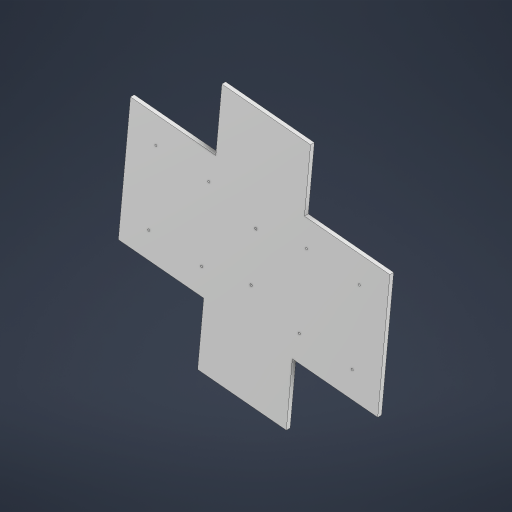
# Autodesk Inventor part: Pod_Holders
Saved by Autodesk Inventor 2024.2 (Build 282272000, 272)
## iProperties
Created: 2024-03-31
Part Number: Pod_Holders
Material: Aluminum
Document SubType Name: Modeling
Designer: warm
Density: 2.7 g/cm^3
Appearance: Satin
Mass: 2143.16 g
Surface Area: 2616.28 cm^2
Volume: 793.761 cm^3
Author: warm
Autodesk Inventor part; units mm, degrees
ref_plane "YZ Plane" through (0, 0, 0) normal (1, 0, 0) x (0, 1, 0)
ref_plane "XZ Plane" through (0, 0, 0) normal (0, 1, 0) x (-1, 0, 0)
sketch "Sketch1" plane through (0, 0, 0) normal (0, 0, 1) x (1, 0, 0)
  line L0 (-65.7194, 60.3542) -> (-75.7574, -47.1434) projected
  line L1 (-75.7574, -47.1434) -> (65.7194, -60.3542) projected
  line L2 (-95.8276, -262.0778) -> (45.6492, -275.2887) projected
  line L3 (-105.8656, -369.5754) -> (-95.8276, -262.0778) projected
  line L4 (-212.6955, 74.0786) -> (-222.7334, -33.419) projected
  line L5 (-222.7334, -33.419) -> (-364.2102, -20.2081) projected
  line L6 (-242.8036, -248.3534) -> (-384.2805, -235.1426) projected
  line L7 (-252.8416, -355.851) -> (-242.8036, -248.3534) projected
  circle A0 centre (-72.4386, -92.2695) radius 2.6 construction
  circle A1 centre (-84.3392, -219.7151) radius 2.6 construction
  circle A2 centre (3.2796, -227.8968) radius 2.6 construction
  circle A3 centre (15.1803, -100.4512) radius 2.6 construction
  circle A4 centre (-156.3158, -105.5656) radius 1.7526 construction
  circle A5 centre (-164.2553, -190.5905) radius 1.7526 construction
  circle A6 centre (-246.2503, -204.5961) radius 2.6 construction
  circle A7 centre (-333.8691, -196.4144) radius 2.6 construction
  circle A8 centre (-321.9685, -68.9688) radius 2.6 construction
  circle A9 centre (-234.3496, -77.1505) radius 2.6 construction
  circle A10 centre (15.1803, -100.4512) radius 1.6
  circle A11 centre (3.2796, -227.8968) radius 1.6
  circle A12 centre (-84.3392, -219.7151) radius 1.6
  circle A13 centre (-72.4386, -92.2695) radius 1.6
  circle A14 centre (-234.3496, -77.1505) radius 1.6
  circle A15 centre (-321.9685, -68.9688) radius 1.6
  circle A16 centre (-333.8691, -196.4144) radius 1.6
  circle A17 centre (-246.2503, -204.5961) radius 1.6
  line L8 (-65.7194, 60.3542) -> (-212.6955, 74.0786)
  line L9 (-364.2102, -20.2081) -> (-384.2805, -235.1426)
  line L10 (-252.8416, -355.851) -> (-105.8656, -369.5754)
  line L11 (45.6492, -275.2887) -> (65.7194, -60.3542)
  circle A18 centre (-156.3158, -105.5656) radius 1.8288
  circle A19 centre (-164.2553, -190.5905) radius 1.8288
  point P0 (0, 0)
  dimension "d0" = 3.2
  dimension "d1" = 3.2
  dimension "d2" = 3.2
  dimension "d3" = 3.2
  dimension "d4" = 3.2
  dimension "d5" = 3.2
  dimension "d6" = 3.2
  dimension "d7" = 3.2
  dimension "d8" = 3.6576
  dimension "d9" = 3.6576
  constraints: 10 centre point, 10 coincident, 8 end point, 3 perpendicular
  measures "d0" diameter of A10
  measures "d1" diameter of A11
  measures "d2" diameter of A12
  measures "d3" diameter of A13
  measures "d4" diameter of A14
  measures "d5" diameter of A15
  measures "d6" diameter of A16
  measures "d7" diameter of A17
  measures "d8" diameter of A18
  measures "d9" diameter of A19
ref_plane "Work Plane1" through (-97.3094, -87.3563, -6.35) normal (0, 0, -1) x (0, 1, 0)
extrude "Extrusion1" add sketch "Sketch1" against normal up to surface (6.35 mm away)
body "Solid1"
